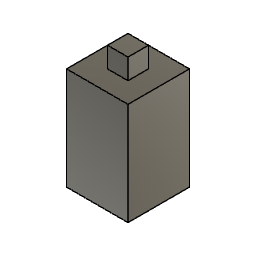
petit_pillier (Autodesk Fusion 360 design; units mm, degrees)
Autodesk Fusion 360 part; units mm, degrees
sketch "Esquisse1" plane through (0, 0, 82) normal (0, 0, 1) x (-1, 0, 0)
  line L0 (200, -190) -> (200, -185)
  line L1 (200, -185) -> (205, -185)
  line L2 (205, -185) -> (205, -190)
  line L3 (205, -190) -> (200, -190)
  line L4 (105, -190) -> (105, -185)
  line L5 (105, -185) -> (110, -185)
  line L6 (110, -185) -> (110, -190)
  line L7 (110, -190) -> (105, -190)
  line L8 (105, -240) -> (105, -235)
  line L9 (105, -235) -> (110, -235)
  line L10 (110, -235) -> (110, -240)
  line L11 (110, -240) -> (105, -240)
  line L12 (200, -240) -> (200, -235)
  line L13 (200, -235) -> (205, -235)
  line L14 (205, -235) -> (205, -240)
  line L15 (205, -240) -> (200, -240)
  line L16 (65, -85) -> (65, -90)
  line L17 (65, -90) -> (60, -90)
  line L18 (60, -90) -> (60, -85)
  line L19 (60, -85) -> (65, -85)
  line L20 (65, -235) -> (65, -240)
  line L21 (65, -240) -> (60, -240)
  line L22 (60, -240) -> (60, -235)
  line L23 (60, -235) -> (65, -235)
  line L24 (250, -235) -> (250, -240)
  line L25 (250, -240) -> (245, -240)
  line L26 (245, -240) -> (245, -235)
  line L27 (245, -235) -> (250, -235)
  line L28 (250, -85) -> (250, -90)
  line L29 (250, -90) -> (245, -90)
  line L30 (245, -90) -> (245, -85)
  line L31 (245, -85) -> (250, -85)
  line L32 (50, -75) -> (50, -250)
  line L33 (50, -250) -> (260, -250)
  line L34 (260, -250) -> (260, -75)
  line L35 (260, -75) -> (50, -75)
  line L36 (156.2462, -202.2177) -> (141.2462, -202.2177)
  line L37 (141.2462, -202.2177) -> (141.2462, -187.2177)
  line L38 (141.2462, -187.2177) -> (156.2462, -187.2177)
  line L39 (156.2462, -187.2177) -> (156.2462, -202.2177)
  dimension "d298" = 15
  dimension "d299" = 15
  constraint horizontal L36
  constraint vertical L37
  constraint horizontal L38
  constraint vertical L39
  measures "d298" distance of L36.start L36.end
  measures "d299" distance of L36.end L37.end
extrude "Extrusion1" add sketch "Esquisse1" along normal blind 25 contours L36 L37 L38 L39
sketch "Esquisse2" plane through (0, 0, 107) normal (0, 0, 1) x (-1, 0, 0)
  line L0 (156.2462, -187.2177) -> (141.2462, -187.2177)
  line L1 (141.2462, -187.2177) -> (141.2462, -202.2177)
  line L2 (141.2462, -202.2177) -> (156.2462, -202.2177)
  line L3 (156.2462, -202.2177) -> (156.2462, -187.2177)
  line L4 (151.2462, -197.2177) -> (146.2462, -197.2177)
  line L5 (146.2462, -197.2177) -> (146.2462, -192.2177)
  line L6 (146.2462, -192.2177) -> (151.2462, -192.2177)
  line L7 (151.2462, -192.2177) -> (151.2462, -197.2177)
  dimension "d302" = 5
  dimension "d303" = 5
  dimension "d304" = 5
  dimension "d305" = 5
  constraint horizontal L4
  constraint vertical L5
  constraint horizontal L6
  constraint vertical L7
  measures "d302" distance of L4.start L4.end
  measures "d303" distance of L4.end L5.end
  measures "d304" distance of L1 L5
  measures "d305" distance of L0 L6
extrude "Extrusion2" add sketch "Esquisse2" along normal blind 5 contours L4 L5 L6 L7
sketch "Esquisse3" plane through (0, 0, 82) normal (0, 0, -1) x (1, 0, 0)
  line L0 (-141.2462, -187.2177) -> (-156.2462, -187.2177)
  line L1 (-156.2462, -187.2177) -> (-156.2462, -202.2177)
  line L2 (-156.2462, -202.2177) -> (-141.2462, -202.2177)
  line L3 (-141.2462, -202.2177) -> (-141.2462, -187.2177)
  line L4 (-151.2462, -192.2177) -> (-146.2462, -192.2177)
  line L5 (-146.2462, -192.2177) -> (-146.2462, -197.2177)
  line L6 (-146.2462, -197.2177) -> (-151.2462, -197.2177)
  line L7 (-151.2462, -197.2177) -> (-151.2462, -192.2177)
  dimension "d308" = 5
  dimension "d309" = 5
  dimension "d310" = 5
  dimension "d311" = 5
  constraint horizontal L4
  constraint vertical L5
  constraint horizontal L6
  constraint vertical L7
  measures "d308" distance of L4.start L4.end
  measures "d309" distance of L4.end L5.end
  measures "d310" distance of L3 L5
  measures "d311" distance of L2 L6
extrude "Extrusion3" add sketch "Esquisse3" along normal blind 5 contours L4 L5 L6 L7
